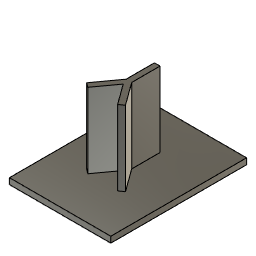
led-lamp-arduino-cover (Autodesk Fusion 360 design; units mm, degrees)
Autodesk Fusion 360 part; units mm, degrees
sketch "Sketch1" plane through (0, 0, 0) normal (0, 0, 1) x (1, 0, 0)
  line L0 (-33.85, 45.35) -> (33.85, 45.35)
  line L1 (33.85, 45.35) -> (33.85, -45.35)
  line L2 (33.85, -45.35) -> (-33.85, -45.35)
  line L3 (-33.85, -45.35) -> (-33.85, 45.35)
  line L4 (0, 0) -> (-33.85, 0)
  line L5 (0, 0) -> (0, 45.35)
  dimension "d13" = 90.7
  dimension "d14" = 67.7
  constraint horizontal L0
  constraint vertical L1
  constraint horizontal L2
  constraint vertical L3
  constraint coincident L4.start L5.start
  constraint midpoint L3 L4.end
  constraint midpoint L0 L5.end
  constraint perpendicular L0 L5
  constraint perpendicular L3 L4
  measures "d13" distance of L0 L2
  measures "d14" distance of L0.start L0.end
extrude "Extrude1" add sketch "Sketch1" along normal blind 4
sketch "Sketch3" plane through (0, 0, 4) normal (0, 0, 1) x (-1, 0, 0)
  line L0 (1.875, -19.5) -> (-1.875, -19.5)
  line L1 (-1.875, -19.5) -> (-1.875, -0.6092)
  line L2 (-1.875, -0.6092) -> (-12.9787, 14.6737)
  line L3 (-12.9787, 14.6737) -> (-9.9449, 16.8779)
  line L4 (-9.9449, 16.8779) -> (0, 3.1899)
  line L5 (0, 3.1899) -> (9.9449, 16.8779)
  line L6 (9.9449, 16.8779) -> (12.9787, 14.6737)
  line L7 (12.9787, 14.6737) -> (1.875, -0.6092)
  line L8 (1.875, -0.6092) -> (1.875, -19.5)
  line L9 (0, -19.5) -> (0, 0)
  line L10 (0, 0) -> (-11.4618, 15.7758)
  line L11 (11.4618, 15.7758) -> (0, 0)
  line L12 (33.85, 45.35) -> (-33.85, 45.35)
  line L13 (-33.85, 45.35) -> (-33.85, -45.35)
  line L14 (-33.85, -45.35) -> (33.85, -45.35)
  line L15 (33.85, -45.35) -> (33.85, 45.35)
  dimension "d7" = 144
  dimension "d8" = 144
  dimension "d9" = 3.75
  dimension "d10" = 19.5
  constraint horizontal L0
  constraint parallel L1 L8
  constraint parallel L2 L4
  constraint parallel L5 L7
  constraint midpoint L0 L9.start
  constraint coincident L9.end L10.start
  constraint midpoint L3 L10.end
  constraint midpoint L6 L11.start
  constraint perpendicular L0 L9
  constraint perpendicular L3 L10
  constraint perpendicular L6 L11
  constraint parallel L4 L10
  constraint parallel L1 L9
  constraint parallel L7 L11
  constraint equal L3 L6
  constraint equal L0 L3
  constraint equal L9 L10
  constraint equal L10 L11
  measures "d7" angle of L9 L10
  measures "d8" angle of L9 L11
  measures "d9" distance of L5.end L6.end
  measures "d10" distance of L9.start L9.end
extrude "Extrude3" add sketch "Sketch3" along normal blind 50 contours L0 L6 L7 L8 L9 L11 | L0 L1 L2 L3 L9 L10 | L3 L4 L5 L6 L10 L11
